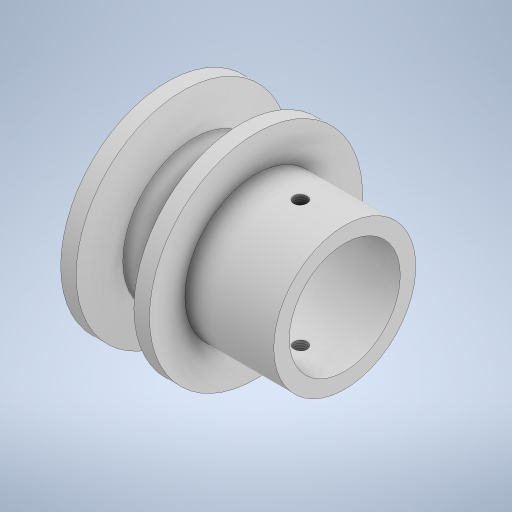
# Autodesk Inventor part: 17701729.303661.004
Saved by Autodesk Inventor 2023 (Build 270158000, 158)
## iProperties
Created: 2022-05-01
Part Number: 17701729.303661.004
Material: Типовые
Document SubType Name: Modeling
Designer: User
Density: 1 g/cm^3
Appearance: По умолчанию
Author: User
Title: Шкив
Autodesk Inventor part; units mm, degrees
ref_plane "YZ Plane" through (0, 0, 0) normal (1, 0, 0) x (0, 1, 0)
ref_plane "XZ Plane" through (0, 0, 0) normal (0, 1, 0) x (-1, 0, 0)
ref_plane "XY Plane" through (0, 0, 0) normal (0, 0, 1) x (1, 0, 0)
sketch "Эскиз1" plane through (0, 0, 0) normal (0, 1, 0) x (-1, 0, 0)
  line L0 (0, 24) -> (20, 24)
  line L1 (20, 24) -> (20, 0)
  line L2 (20, 0) -> (0, 0)
  line L3 (20, 24) -> (14, 24)
  line L4 (14, 16) -> (6, 16)
  line L5 (20, 0) -> (-20, 0)
  line L6 (-20, 0) -> (-20, 16)
  line L7 (-20, 16) -> (0, 16)
  line L8 (-20, 0) -> (-20, 12.5)
  line L9 (0, 16) -> (0, 24)
  line L10 (10, 24) -> (3.5, 24)
  line L11 (3.5, 24) -> (6, 16)
  line L12 (3.5, 24) -> (16.5, 24)
  line L13 (16.5, 24) -> (14, 16)
  line L14 (20, 0) -> (20, 16.5)
  line L15 (0, 0) -> (5, 0)
  line L16 (0, 16) -> (5, 16)
  line L17 (-20, 12.5) -> (5, 12.5)
  line L18 (5, 12.5) -> (20, 12.5)
  point P0 (16.5, 24)
  point P1 (20, 20.5)
  dimension "d0" = 24
  dimension "d1" = 20
  dimension "d3" = 8
  dimension "d5" = 40
  dimension "d6" = 16
  dimension "d7" = 12.5
  dimension "d15" = 6.5
  dimension "d16" = 13
  constraints: 38 end point, 9 point on line, 6 perpendicular, 1 midpoint, 1 vertical
  measures "d0" distance of L2.end L0.start
  measures "d1" distance of L0.start L0.end
  measures "d3" distance of L3.end L4.start
  measures "d5" distance of L1.end L5.end
  measures "d6" distance of L5.end L6.end
  measures "d7" distance of L5.end L8.end
  measures "d15" distance of L10.start L10.end
  measures "d16" distance of L10.end L12.end
revolve "Вращение4" add sketch "Эскиз1" angle 360 about axis through (-20, 0, 0) along (1, 0, 0) contours L0 L11 L4 L13 L1 L18 L17 L6 L7 L9
sketch "Эскиз4" plane through (0, 0, 0) normal (0, 1, 0) x (-1, 0, 0)
  line L0 (-20, 16) -> (-20, -16) projected
  line L1 (-20, 0) -> (0, 0)
  line L2 (0, 0) -> (-10, 0)
  circle A0 centre (-10, 0) radius 1.5
  dimension "d43" = 3
  constraints: 4 end point, 2 midpoint, 1 centre point, 1 coincident, 1 horizontal
  measures "d43" diameter of A0
extrude "Выдавливание5" cut sketch "Эскиз4" along normal mid plane 59.25
thread "Резьба4" size "M3x0.5" class "6H" standard "ANSI Metric M Profile" full length
